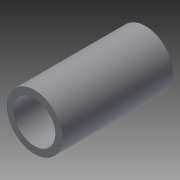
# Autodesk Inventor part: M - 0.375 Aluminum Tube Spacer
Saved by Autodesk Inventor 2013 (Build 170138000, 138)
## iProperties
Created: 2013-02-17
Part Number: M - 0.375 Aluminum Tube Spacer
Material: Generic
Document SubType Name: Modeling
Designer: Moses
Density: 1 g/cm^3
Mass: 1.4077 g
Surface Area: 18.8432 cm^2
Volume: 1.4077 cm^3
Author: Moses
Autodesk Inventor part; units mm, degrees
ref_plane "YZ Plane" through (0, 0, 0) normal (1, 0, 0) x (0, 1, 0)
ref_plane "XZ Plane" through (0, 0, 0) normal (0, 1, 0) x (-1, 0, 0)
ref_plane "XY Plane" through (0, 0, 0) normal (0, 0, 1) x (1, 0, 0)
sketch "Sketch1" plane through (0, 0, 0) normal (0, 0, 1) x (1, 0, 0)
  circle A0 centre (0, 0) radius 4.7625
  circle A1 centre (0, 0) radius 6.35
  dimension "d0" = 9.525
  dimension "d2" = 12.7
  constraints: 2 centre point, 2 coincident
  measures "d0" diameter of A0
  measures "d2" diameter of A1
extrude "Extrusion1" add sketch "Sketch1" along normal blind 25.4
body "Solid1"
